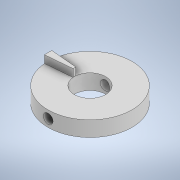
# Autodesk Inventor part: 10d_coupler
Saved by Autodesk Inventor 2021 (Build 250183000, 183)
## iProperties
Created: 2024-02-08
Part Number: 10d_coupler
Material: Generic
Document SubType Name: Modeling
Designer: Sebastián
Density: 1 g/cm^3
Appearance: Default
Author: Sebastián
Autodesk Inventor part; units mm, degrees
ref_plane "YZ Plane" through (0, 0, 0) normal (1, 0, 0) x (0, 1, 0)
ref_plane "XZ Plane" through (0, 0, 0) normal (0, 1, 0) x (-1, 0, 0)
ref_plane "XY Plane" through (0, 0, 0) normal (0, 0, 1) x (1, 0, 0)
sketch "Sketch1" plane through (0, 0, 0) normal (0, 1, 0) x (-1, 0, 0)
  circle A0 centre (0, 0) radius 4.1
  circle A1 centre (0, 0) radius 11
  dimension "d0" = 8.2
  dimension "d1" = 22
  constraints: 2 centre point, 2 coincident
  measures "d0" diameter of A0
  measures "d1" diameter of A1
extrude "Extrusion1" add sketch "Sketch1" along normal blind 4
sketch "Sketch2" plane through (0, 4, 0) normal (0, 1, 0) x (1, 0, 0)
  line L0 (0, 0) -> (-8.1688, -0.7147) construction
  line L1 (0, 0) -> (-8.1688, 0.7147) construction
  arc A0 (-4.0844, 0.3573) -> (-4.0844, -0.3573) centre (10.5368, 0) ccw
  line L2 (-4.0844, 0.3573) -> (-10.9581, 0.9587)
  line L3 (-15.4, 0) -> (15.4, 0) construction
  circle A1 centre (0, 0) radius 4.1 construction
  circle A2 centre (0, 0) radius 11 construction
  line L4 (-4.0844, -0.3573) -> (-10.9581, -0.9587)
  circle A3 centre (0, 0) radius 11 projected
  dimension "d4" = 10
  constraints: 8 end point, 3 point on circle, 2 midpoint, 1 centre point, 1 coincident, 1 collinear, 1 point on line, 1 symmetric about line, 4 other
  measures "d4" angle of L1 L0
extrude "Extrusion2" add sketch "Sketch2" along normal blind 2 contours A0 L4 A3 L2 picked at (-8.693, 0.0397)
sketch "Sketch3" plane through (0, 0, 0) normal (0, 0, 1) x (1, 0, 0)
  circle A0 centre (0, 2) radius 1.25
  line L0 (11, 0) -> (-11, 0) projected
  point P0 (0, 0)
  dimension "d7" = 2.5
  dimension "d8" = 2
  constraints: 1 centre point
  measures "d7" diameter of A0
  measures "d8" distance from line of L0 A0.centre
extrude "Extrusion3" cut sketch "Sketch3" against normal through all both and the other way through all
body "Solid1"
